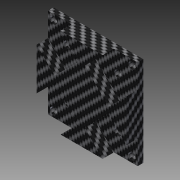
# Autodesk Inventor part: top
Saved by Autodesk Inventor 2015 (Build 190159000, 159)
## iProperties
Created: 2016-11-27
Part Number: top
Material: Generic
Document SubType Name: Modeling
Designer: Hampus
Density: 1 g/cm^3
Appearance: Carbon Fiber
Author: Hampus
Autodesk Inventor part; units mm, degrees
ref_plane "YZ Plane" through (0, 0, 0) normal (1, 0, 0) x (0, 1, 0)
ref_plane "XZ Plane" through (0, 0, 0) normal (0, 1, 0) x (-1, 0, 0)
ref_plane "XY Plane" through (0, 0, 0) normal (0, 0, 1) x (1, 0, 0)
sketch "Sketch1" plane through (0, 0, 0) normal (0, 1, 0) x (-1, 0, 0)
  line L0 (0, -32) -> (-32, -32)
  line L1 (-32, -32) -> (-32, 0)
  line L2 (-32, 0) -> (0, 0)
  line L3 (0, 0) -> (0, -32)
  line L4 (0, 0) -> (-4, 0)
  line L5 (-32, 0) -> (-32, -4)
  circle A0 centre (-2, -2) radius 1.25
  circle A1 centre (-30, -2) radius 1.25
  circle A2 centre (-2, -30) radius 1.25
  circle A3 centre (-30, -30) radius 1.25
  line L6 (0, -32) -> (65, -32) construction
  line L7 (-32, -32) -> (33, -32) construction
  line L8 (-8.4853, -32) -> (-14.8492, -25.636)
  line L9 (0, -23.5147) -> (-6.364, -17.1508)
  line L10 (-6.364, -17.1508) -> (-14.8492, -25.636)
  circle A4 centre (-7.0711, -24.9289) radius 1.25
  line L11 (-23.5147, -32) -> (-17.1508, -25.636)
  line L12 (-32, -23.5147) -> (-25.636, -17.1508)
  line L13 (-25.636, -17.1508) -> (-17.1508, -25.636)
  circle A5 centre (-24.9289, -24.9289) radius 1.25
  line L14 (-8.4853, 0) -> (-14.8492, -6.364)
  line L15 (0, -8.4853) -> (-6.364, -14.8492)
  line L16 (-6.364, -14.8492) -> (-14.8492, -6.364)
  circle A6 centre (-7.0711, -7.0711) radius 1.25
  line L17 (-23.5147, 0) -> (-17.1508, -6.364)
  line L18 (-32, -8.4853) -> (-25.636, -14.8492)
  circle A7 centre (-24.9289, -7.0711) radius 1.25
  line L19 (-25.636, -14.8492) -> (-17.1508, -6.364)
  point P0 (0, 0)
  dimension "d8" = 4
  dimension "d10" = 2.5
  dimension "d11" = 2.5
  constraints: 40 end point, 11 point on line, 8 centre point, 2 horizontal, 2 parallel, 1 perpendicular
  measures "d8" distance of L1.end L5.end
  measures "d10" diameter of A0
  measures "d11" diameter of A1
extrude "Extrusion1" add sketch "Sketch1" along normal blind 6
extrude "Extrusion2" cut sketch "Sketch1" along normal blind 4 contours L0 L8 L10 L9 L3 | L0 L1 L12 L13 L11 | L15 L16 L14 L2 L3 | L1 L2 L17 L19 L18
body "Solid1"
